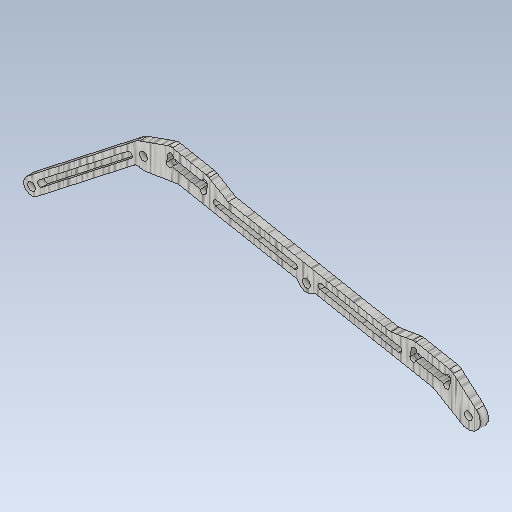
# Autodesk Inventor part: 台形サスバー２
Saved by Autodesk Inventor 2020 (Build 240168000, 168)
## iProperties
Created: 2019-11-14
Part Number: 台形サスバー２
Material: アルミニウム 7075
Document SubType Name: Modeling
Designer: tanjihayato
Density: 2.81 g/cm^3
Appearance: サテン - ブラシ仕上げ 重厚
Mass: 9.37217 g
Surface Area: 46.6831 cm^2
Volume: 3.33529 cm^3
Author: tanjihayato
Autodesk Inventor part; units mm, degrees
note: some values were not read from the file. Chosen so that the rebuilt part matches the saved one: sketch regions of "押し出し1".
ref_plane "YZ Plane" through (0, 0, 0) normal (1, 0, 0) x (0, 1, 0)
ref_plane "XZ Plane" through (0, 0, 0) normal (0, 1, 0) x (-1, 0, 0)
ref_plane "XY Plane" through (0, 0, 0) normal (0, 0, 1) x (1, 0, 0)
sketch "スケッチ1" plane through (0, 0, 0) normal (0, 0, 1) x (1, 0, 0)
  circle A0 centre (127.64315, 30.26217) radius 1.5
  circle A1 centre (5.936242, 53.5882) radius 1.5
  line L0 (5.936242, 53.5882) -> (127.64315, 30.26217) construction
  circle A2 centre (5.936242, 53.5882) radius 4.025
  circle A3 centre (127.64315, 30.26217) radius 4.025
  arc A4 (127.25169, 23.248085) -> (128.965476, 37.161596) centre (127.64315, 30.26217) ccw
  line L1 (12.835668, 52.265874) -> (13.400362, 55.212248)
  line L2 (15.462824, 54.816962) -> (26.069771, 52.784062)
  line L3 (28.132233, 52.388776) -> (27.567538, 49.442402)
  line L4 (14.89813, 51.870588) -> (25.505076, 49.837688)
  line L5 (120.743724, 31.584496) -> (121.308418, 34.53087)
  line L6 (119.245956, 34.926156) -> (108.63901, 36.959056)
  line L7 (106.576548, 37.354342) -> (106.011853, 34.407968)
  line L8 (108.074315, 34.012682) -> (118.681262, 31.979782)
  circle A5 centre (19.354562, 46.434577) radius 3
  circle A6 centre (112.530747, 28.576671) radius 3
  line L9 (7.258568, 60.487626) -> (128.965476, 37.161596)
  arc A7 (17.926333, 42.16724) -> (21.546529, 42.504529) centre (19.354562, 46.434577) ccw
  arc A8 (109.041036, 25.735559) -> (112.27999, 24.083663) centre (112.530747, 28.576671) ccw
  line L10 (3.706619, 46.926413) -> (17.926333, 42.16724)
  line L11 (112.27999, 24.083663) -> (127.25169, 23.248085)
  circle A9 centre (19.354562, 46.434577) radius 1.5
  circle A10 centre (112.530747, 28.576671) radius 1.5
  line L12 (32.344248, 48.52691) -> (21.546529, 42.504529)
  line L13 (109.041036, 25.735559) -> (101.235144, 35.32346)
  line L14 (32.344248, 48.52691) -> (101.235144, 35.32346)
  arc A11 (108.63901, 36.959056) -> (106.576548, 37.354342) centre (107.607779, 37.156699) ccw
  arc A12 (106.011853, 34.407968) -> (108.074315, 34.012682) centre (107.043084, 34.210325) ccw
  arc A13 (121.308418, 34.53087) -> (119.245956, 34.926156) centre (120.277187, 34.728513) ccw
  arc A14 (118.681262, 31.979782) -> (120.743724, 31.584496) centre (119.712493, 31.782139) ccw
  arc A15 (28.132233, 52.388776) -> (26.069771, 52.784062) centre (27.101002, 52.586419) ccw
  arc A16 (25.505076, 49.837688) -> (27.567538, 49.442402) centre (26.536307, 49.640045) ccw
  arc A17 (15.462824, 54.816962) -> (13.400362, 55.212248) centre (14.431593, 55.014605) ccw
  arc A18 (12.835668, 52.265874) -> (14.89813, 51.870588) centre (13.866899, 52.068231) ccw
  line L15 (5.936242, 53.5882) -> (-35.940425, 22.842004) construction
  circle A19 centre (-35.940425, 22.842004) radius 1.5
  arc A20 (-37.715892, 25.26021) -> (-34.164958, 20.423799) centre (-35.940425, 22.842004) ccw
  line L16 (-37.715892, 25.26021) -> (-0.959545, 52.247024)
  line L17 (-34.164958, 20.423799) -> (2.591389, 47.410613)
  arc A21 (7.258568, 60.487626) -> (-0.959545, 52.247024) centre (5.936242, 53.5882) ccw
  arc A22 (2.591389, 47.410613) -> (3.706619, 46.926413) centre (5.936242, 53.5882) ccw
  point P0 (0, 0)
  point P1 (0, 0)
  dimension "d0" = 8.05
  dimension "d1" = 8.05
  dimension "d2" = 3
  dimension "d3" = 3
  dimension "d4" = 15
  dimension "d5" = 3
  dimension "d6" = 15
  dimension "d7" = 6
  dimension "d8" = 6
  dimension "d9" = 9
  dimension "d10" = 9
  dimension "d11" = 3
  dimension "d12" = 3
  dimension "d13" = 7.5
  dimension "d14" = 7.5
  dimension "d15" = 40
  dimension "d16" = 40
  dimension "d17" = 2.1
  dimension "d18" = 2.1
  dimension "d19" = 2.1
  dimension "d20" = 2.1
  dimension "d21" = 2.1
  dimension "d22" = 2.1
  dimension "d23" = 2.1
  dimension "d24" = 2.1
  dimension "d25" = 3
  dimension "d26" = 6
  dimension "d27" = 3
  dimension "d28" = 3
  constraints: 36 end point, 28 point on circle, 23 centre point, 22 tangent, 14 point on line, 8 coincident, 4 parallel, 4 perpendicular, 1 collinear
  measures "d0" diameter of A2
  measures "d1" diameter of A3
  measures "d2" radial gap between concentric circles of A3 A4
  measures "d3" distance of L1.start L1.end
  measures "d4" distance of L1.end L3.start
  measures "d5" distance of L5.start L5.end
  measures "d6" distance of L5.end L7.start
  measures "d7" diameter of A5
  measures "d8" diameter of A6
  measures "d9" diameter of A7
  measures "d10" diameter of A8
  measures "d11" diameter of A9
  measures "d12" diameter of A10
  measures "d13" distance from line of A5.centre L3
  measures "d14" distance from line of A10.centre L7
  measures "d15" angle of L13 L0
  measures "d16" angle of L0 L12
  measures "d17" diameter of A11
  measures "d18" diameter of A12
  measures "d19" diameter of A13
  measures "d20" diameter of A14
  measures "d21" diameter of A15
  measures "d22" diameter of A16
  measures "d23" diameter of A17
  measures "d24" diameter of A18
  measures "d25" diameter of A19
  measures "d26" diameter of A20
  measures "d27" radial gap between concentric circles of A21 A2
  measures "d28" radial gap between concentric circles of A22 A2
sketch "スケッチ3" plane through (0, 0, 0) normal (0, 0, 1) x (1, 0, 0)
  circle A0 centre (0, 0) radius 10.1 construction
  circle A1 centre (25.320198, -9.936175) radius 17.1 construction
  circle A2 centre (110.474331, -16.4118) radius 28.1 construction
  circle A3 centre (62.413099, -12.756939) radius 20.1 construction
  circle A4 centre (-21.690847, -16.4118) radius 17.1 construction
  circle A5 centre (-105.525669, -16.4118) radius 28.1 construction
  line L0 (-170.91498, -81.4118) -> (490.004419, -81.4118)
  line L1 (-105.525669, -16.4118) -> (-21.690847, -16.4118) construction
  line L2 (110.474331, -16.4118) -> (25.320198, -9.936175) construction
  line L3 (110.474331, -16.4118) -> (104.150058, -0.631953)
  line L4 (104.150058, -0.631953) -> (95.593688, 20.717252) construction
  line L5 (95.593688, 20.717252) -> (70.474331, -10.4118) construction
  line L6 (70.474331, -10.4118) -> (110.474331, -16.4118) construction
  line L7 (-137.681852, 53.5882) -> (165.818568, 53.5882)
  line L8 (25.320198, -9.936175) -> (108.686903, 8.5882) construction
  line L9 (25.320198, -9.936175) -> (102.538646, -46.4118) construction
  line L10 (25.320198, -9.936175) -> (5.936242, 53.5882) construction
  line L11 (5.936242, 53.5882) -> (127.64315, 30.26217)
  line L12 (127.64315, 30.26217) -> (110.474331, -16.4118) construction
  line L13 (102.538646, -46.4118) -> (118.068109, 0.832921) construction
  line L14 (118.068109, 0.832921) -> (5.936242, 53.5882) construction
  line L15 (108.686903, 8.5882) -> (129.858294, 53.5882) construction
  line L16 (129.858294, 53.5882) -> (5.936242, 53.5882) construction
  line L17 (119.272599, 31.0882) -> (366.444098, 68.5882) construction
  line L18 (119.05874, 6.925185) -> (362.021337, 65.824902) construction
  line L19 (110.303378, -22.78944) -> (351.062397, 44.553669) construction
  line L20 (127.64315, 30.26217) -> (4.192658, 19.461651) construction
  circle A6 centre (80.474331, 23.123973) radius 3 construction
  circle A7 centre (80.474331, 23.123973) radius 1.5
  arc A8 (79.800999, 27.573313) -> (76.161969, 24.409872) centre (80.474331, 23.123973) ccw
  circle A9 centre (70.474331, -10.4118) radius 1.5
  arc A10 (66.161969, -9.125901) -> (69.424217, -14.787558) centre (70.474331, -10.4118) ccw
  circle A11 centre (150.474331, 0.5882) radius 1.5
  arc A12 (152.562257, -3.398097) -> (154.040845, 3.33228) centre (150.474331, 0.5882) ccw
  circle A13 centre (127.64315, 30.26217) radius 1.5
  arc A14 (131.281576, 32.91016) -> (126.969818, 34.71151) centre (127.64315, 30.26217) ccw
  circle A15 centre (110.474331, -16.4118) radius 5
  arc A16 (108.607462, -24.190926) -> (114.186199, -23.49855) centre (110.474331, -16.4118) ccw
  line L21 (76.161969, 24.409872) -> (66.161969, -9.125901)
  line L22 (69.424217, -14.787558) -> (108.607462, -24.190926)
  line L23 (114.186199, -23.49855) -> (152.562257, -3.398097)
  line L24 (154.040845, 3.33228) -> (131.209664, 33.00625)
  line L25 (126.969818, 34.71151) -> (79.800999, 27.573313)
  circle A17 centre (-145.525669, 0.5882) radius 1.5
  arc A18 (-149.092184, 3.33228) -> (-147.613596, -3.398097) centre (-145.525669, 0.5882) ccw
  circle A19 centre (-105.525669, -16.4118) radius 5
  arc A20 (-109.237538, -23.49855) -> (-103.6588, -24.190926) centre (-105.525669, -16.4118) ccw
  circle A21 centre (-65.525669, -10.4118) radius 1.5
  arc A22 (-64.475556, -14.787558) -> (-61.213308, -9.125901) centre (-65.525669, -10.4118) ccw
  circle A23 centre (0, 0) radius 20.05 construction
  circle A24 centre (110.474331, -16.4118) radius 30.1 construction
  circle A25 centre (62.413099, -12.756939) radius 22.1 construction
  circle A26 centre (25.320198, -9.936175) radius 19.1 construction
  circle A27 centre (0, 0) radius 12.1 construction
  circle A28 centre (-21.690847, -16.4118) radius 19.1 construction
  circle A29 centre (-105.525669, -16.4118) radius 30.1 construction
  circle A30 centre (0, 0) radius 20.55 construction
  circle A31 centre (95.593688, 20.717252) radius 4.025 construction
  circle A32 centre (95.593688, 20.717252) radius 6.025 construction
  circle A33 centre (-75.525669, 23.123973) radius 1.5
  arc A34 (-71.213308, 24.409872) -> (-74.852338, 27.573313) centre (-75.525669, 23.123973) ccw
  circle A35 centre (-122.694488, 30.26217) radius 1.5
  arc A36 (-122.021157, 34.71151) -> (-126.261003, 33.00625) centre (-122.694488, 30.26217) ccw
  line L26 (-126.261003, 33.00625) -> (-149.092184, 3.33228)
  line L27 (-147.613596, -3.398097) -> (-109.237538, -23.49855)
  line L28 (-103.6588, -24.190926) -> (-64.475556, -14.787558)
  line L29 (-61.213308, -9.125901) -> (-71.213308, 24.409872)
  line L30 (-74.852338, 27.573313) -> (-122.021157, 34.71151)
  circle A37 centre (14, -17.4118) radius 2.29213 construction
  circle A38 centre (-14, -17.4118) radius 2.29213 construction
  circle A39 centre (-14, -17.4118) radius 14 construction
  circle A40 centre (14, -17.4118) radius 14 construction
  line L31 (-170.651239, -31.4118) -> (202.86558, -31.4118)
  line L32 (5.936242, 53.5882) -> (-42.252867, 34.177029) construction
  line L33 (5.936242, 53.5882) -> (-29.404465, 15.509095) construction
  circle A41 centre (5.936242, 53.5882) radius 1.5
  arc A42 (9.961109, 55.600773) -> (4.254869, 57.762285) centre (5.936242, 53.5882) ccw
  line L34 (-21.690847, -16.4118) -> (-99.974162, 13.5882) construction
  line L35 (-21.690847, -16.4118) -> (-101.711328, -41.4118) construction
  line L36 (9.961109, 55.600773) -> (31.415648, 12.694659)
  circle A43 centre (-50.601037, 30.814282) radius 1.5
  arc A44 (-52.28241, 34.988367) -> (-54.424801, 28.441767) centre (-50.601037, 30.814282) ccw
  line L37 (4.254869, 57.762285) -> (-52.28241, 34.988367)
  line L38 (-54.424801, 28.441767) -> (-46.715132, 16.016156)
  circle A45 centre (27.390781, 10.682087) radius 3 construction
  circle A46 centre (-84.86606, 5.271327) radius 4.5 construction
  circle A47 centre (-132.017427, -1.981251) radius 4.5 construction
  line L39 (-132.701548, 2.466443) -> (-85.550181, 9.71902) construction
  arc A48 (26.900287, 6.208898) -> (31.415648, 12.694659) centre (27.390781, 10.682087) ccw
  arc A49 (-46.715132, 16.016156) -> (-43.381863, 13.915483) centre (-42.891368, 18.388671) ccw
  line L40 (-43.381863, 13.915483) -> (26.900287, 6.208898)
  circle A50 centre (-42.252867, 34.177029) radius 3 construction
  circle A51 centre (25.320198, -9.936175) radius 4.025 construction
  circle A52 centre (-21.690847, -16.4118) radius 4.025 construction
  circle A53 centre (-42.891368, 18.388671) radius 1.5
  circle A54 centre (27.390781, 10.682087) radius 1.5
  circle A55 centre (-57.813011, 39.770535) radius 4.5 construction
  circle A56 centre (-99.303951, 63.315241) radius 4.5 construction
  line L41 (5.936242, 53.5882) -> (-35.940425, 22.842004) construction
  circle A57 centre (-58.005574, -24.479052) radius 20.1 construction
  circle A58 centre (-58.005574, -24.479052) radius 22.1 construction
  line L42 (-53.326057, 39.428119) -> (-56.279689, 0.724331) construction
  circle A59 centre (-42.252867, 34.177029) radius 4.5
  dimension "d14" = 7.5
  dimension "d125" = 9
  dimension "d126" = 9
  dimension "d141" = 9
  dimension "d37" = 20.2
  dimension "d38" = 34.2
  dimension "d39" = 56.2
  dimension "d40" = 40.2
  dimension "d41" = 216
  dimension "d42" = 65
  dimension "d43" = 65
  dimension "d44" = 34.2
  dimension "d45" = 56.2
  dimension "d46" = 17
  dimension "d47" = 23
  dimension "d48" = 40
  dimension "d49" = 40
  dimension "d50" = 6
  dimension "d51" = 135
  dimension "d52" = 25
  dimension "d53" = 30
  dimension "d54" = 5
  dimension "d55" = 2
  dimension "d56" = 250
  dimension "d57" = 150
  dimension "d58" = 250
  dimension "d59" = 250
  dimension "d60" = 123.823
  dimension "d61" = 123.823
  dimension "d62" = 123.823
  dimension "d63" = 6
  dimension "d64" = 3
  dimension "d65" = 9
  dimension "d66" = 3
  dimension "d67" = 9
  dimension "d68" = 3
  dimension "d69" = 9
  dimension "d70" = 40
  dimension "d71" = 17
  dimension "d72" = 3
  dimension "d73" = 9
  dimension "d74" = 10
  dimension "d75" = 3
  dimension "d76" = 3
  dimension "d77" = 9
  dimension "d78" = 40
  dimension "d79" = 17
  dimension "d80" = 10
  dimension "d81" = 3
  dimension "d82" = 3
  dimension "d83" = 9
  dimension "d84" = 40
  dimension "d85" = 6
  dimension "d86" = 40.1
  dimension "d87" = 2
  dimension "d88" = 2
  dimension "d89" = 2
  dimension "d90" = 2
  dimension "d91" = 2
  dimension "d92" = 2
  dimension "d93" = 0.5
  dimension "d94" = 8.05
  dimension "d95" = 2
  dimension "d96" = 3
  dimension "d97" = 9
  dimension "d98" = 3
  dimension "d99" = 9
  dimension "d100" = 46.67397
  constraints: 86 end point, 57 centre point, 39 tangent, 29 coincident, 29 point on circle, 11 equal length, 5 horizontal, 3 midpoint, 3 point on line, 2 equal radius, 1 collinear, 1 parallel, 1 perpendicular, 13 other
  measures "d37" diameter of A0
  measures "d38" diameter of A1
  measures "d39" diameter of A2
  measures "d40" diameter of A3
  measures "d41" distance of L1.start L2.start
  measures "d42" distance from line of L0 L2.start
  measures "d43" distance from line of L0 L1.start
  measures "d44" diameter of A4
  measures "d45" diameter of A5
  measures "d46" distance of L2.start L3.end
  measures "d47" distance of L3.end L4.end
  measures "d48" distance of L4.end L5.end
  measures "d49" horizontal distance of L5.end L2.start
  measures "d50" vertical distance of L5.end L2.start
  measures "d51" distance between parallel lines of L0 L7
  measures "d52" vertical distance of L2.start L8.end
  measures "d53" vertical distance of L9.end L2.start
  measures "d54" angle of L12 L15
  measures "d55" angle of L12 L13
  measures "d56" distance of L17.start L17.end
  measures "d57" distance from line of L0 L17.end
  measures "d58" distance of L18.start L18.end
  measures "d59" distance of L19.start L19.end
  measures "d60" angle of L15 L17
  measures "d61" angle of L12 L18
  measures "d62" angle of L13 L19
  measures "d63" diameter of A6
  measures "d64" diameter of A7
  measures "d65" diameter of A8
  measures "d66" diameter of A9
  measures "d67" diameter of A10
  measures "d68" diameter of A11
  measures "d69" diameter of A12
  measures "d70" horizontal distance of L2.start A11.centre
  measures "d71" vertical distance of L2.start A11.centre
  measures "d72" diameter of A13
  measures "d73" diameter of A14
  measures "d74" diameter of A15
  measures "d75" radial gap between concentric circles of A15 A16
  measures "d76" diameter of A17
  measures "d77" diameter of A18
  measures "d78" horizontal distance of L1.start A17.centre
  measures "d79" vertical distance of L1.start A18.centre
  measures "d80" diameter of A19
  measures "d81" radial gap between concentric circles of A19 A20
  measures "d82" diameter of A21
  measures "d83" diameter of A22
  measures "d84" horizontal distance of L1.start A21.centre
  measures "d85" vertical distance of L1.start A21.centre
  measures "d86" diameter of A23
  measures "d87" radial gap between concentric circles of A2 A24
  measures "d88" radial gap between concentric circles of A3 A25
  measures "d89" radial gap between concentric circles of A1 A26
  measures "d90" radial gap between concentric circles of A0 A27
  measures "d91" radial gap between concentric circles of A4 A28
  measures "d92" radial gap between concentric circles of A5 A29
  measures "d93" radial gap between concentric circles of A23 A30
  measures "d94" diameter of A31
  measures "d95" radial gap between concentric circles of A31 A32
  measures "d96" diameter of A33
  measures "d97" diameter of A34
  measures "d98" diameter of A35
  measures "d99" diameter of A36
  measures "d100" vertical distance of L2.start L11.end
sketch "スケッチ2" plane through (0, 0, 0) normal (0, 0, 1) x (1, 0, 0)
  circle A0 centre (-35.940425, 22.842004) radius 1.5
  circle A1 centre (5.936242, 53.5882) radius 1.5
  circle A2 centre (127.64315, 30.26217) radius 1.5
  line L0 (19.061011, 51.072741) -> (114.518381, 32.777629)
  circle A3 centre (5.936242, 53.5882) radius 4.5
  circle A4 centre (127.64315, 30.26217) radius 4.5
  circle A5 centre (-35.940425, 22.842004) radius 3
  line L1 (5.0892, 49.168639) -> (6.071325, 48.980408)
  line L2 (6.071325, 48.980408) -> (19.061011, 51.072741)
  line L3 (114.518381, 32.777629) -> (125.813983, 26.03084)
  line L4 (125.813983, 26.03084) -> (126.796108, 25.842609)
  line L5 (4.441871, 57.832827) -> (15.204741, 61.622021)
  line L6 (-37.784972, 25.207939) -> (3.169421, 57.137102)
  line L7 (3.512579, 49.796649) -> (-34.095878, 20.47607)
  line L8 (122.00181, 41.153572) -> (130.601007, 33.653494)
  circle A6 centre (80.318062, 36.277771) radius 3
  circle A7 centre (80.318062, 36.277771) radius 4.5
  line L9 (128.210589, 34.72625) -> (80.885502, 40.741852)
  circle A8 centre (80.474331, 23.123973) radius 1.5
  line L10 (120.463576, 35.710991) -> (121.028271, 38.657365)
  line L11 (15.186361, 58.942751) -> (14.621667, 55.996377)
  circle A9 centre (66.977927, 42.90731) radius 1.5
  circle A10 centre (66.977927, 42.90731) radius 3
  line L12 (29.918232, 56.119279) -> (29.353537, 53.172905)
  arc A11 (17.248823, 58.547465) -> (15.186361, 58.942751) centre (16.217592, 58.745108) ccw
  arc A12 (29.918232, 56.119279) -> (27.85577, 56.514565) centre (28.887001, 56.316922) ccw
  arc A13 (27.291076, 53.568191) -> (29.353537, 53.172905) centre (28.322307, 53.370548) ccw
  arc A14 (14.621667, 55.996377) -> (16.684129, 55.601091) centre (15.652898, 55.798734) ccw
  line L13 (17.248823, 58.547465) -> (27.85577, 56.514565)
  line L14 (16.684129, 55.601091) -> (27.291076, 53.568191)
  arc A15 (31.882481, 55.742816) -> (27.00191, 58.714615) centre (28.887001, 56.316922) ccw
  line L15 (27.00191, 58.714615) -> (18.855609, 60.275914)
  arc A16 (18.855609, 60.275914) -> (15.204741, 61.622021) centre (16.217592, 58.745108) ccw
  line L16 (106.2964, 41.480837) -> (105.731706, 38.534463)
  arc A17 (108.358862, 41.085551) -> (106.2964, 41.480837) centre (107.327631, 41.283194) ccw
  arc A18 (121.028271, 38.657365) -> (118.965809, 39.052651) centre (119.99704, 38.855008) ccw
  arc A19 (118.401114, 36.106277) -> (120.463576, 35.710991) centre (119.432345, 35.908634) ccw
  arc A20 (105.731706, 38.534463) -> (107.794168, 38.139177) centre (106.762937, 38.33682) ccw
  line L17 (31.882481, 55.742816) -> (104.332151, 41.8573)
  line L18 (108.358862, 41.085551) -> (118.965809, 39.052651)
  line L19 (107.794168, 38.139177) -> (118.401114, 36.106277)
  arc A21 (122.00181, 41.153572) -> (118.111949, 41.252701) centre (119.99704, 38.855008) ccw
  line L20 (118.111949, 41.252701) -> (109.965648, 42.814)
  arc A22 (109.965648, 42.814) -> (104.332151, 41.8573) centre (107.327631, 41.283194) ccw
  line L21 (30.450999, 58.935397) -> (37.645199, 54.638348)
  line L22 (16.791698, 61.740588) -> (29.461109, 59.312402)
  line L23 (120.571146, 41.850488) -> (107.901737, 44.278674)
  line L24 (106.8426, 44.294381) -> (98.569433, 42.961768)
  point P0 (0, 0)
  dimension "d36" = 9
  dimension "d29" = 9
  dimension "d30" = 9
  dimension "d31" = 6
  dimension "d35" = 6
  dimension "d155" = 47.70588
  dimension "d156" = 47.70588
  dimension "d163" = 3
  dimension "d164" = 3
  dimension "d166" = 8.07688
  dimension "d167" = 8.07688
  dimension "d168" = 3
  dimension "d169" = 6
  dimension "d170" = 61.9691
  dimension "d171" = 61.9691
  dimension "d174" = 15
  dimension "d175" = 2.1
  dimension "d176" = 2
  dimension "d178" = 2
  dimension "d179" = 2
  dimension "d180" = 15
  dimension "d181" = 2.1
  dimension "d182" = 7
  dimension "d183" = 2
  dimension "d184" = 2
  dimension "d187" = 160
  dimension "d188" = 160
  dimension "d189" = 160
  dimension "d190" = 160
  dimension "d191" = 1
  dimension "d192" = 1
  constraints: 50 end point, 39 point on circle, 26 tangent, 18 centre point, 13 point on line, 9 perpendicular, 7 parallel, 6 equal radius, 5 coincident, 2 collinear, 5 other
  measures "d29" diameter of A3
  measures "d30" diameter of A4
  measures "d31" diameter of A5
  measures "d35" diameter of A6
  measures "d155" distance of A8.centre A2.centre
  measures "d156" distance of A2.centre A6.centre
  measures "d163" distance of L10.start L10.end
  measures "d164" distance of L11.start L11.end
  measures "d166" distance from line of A2.centre L10
  measures "d167" distance from line of A1.centre L11
  measures "d168" diameter of A9
  measures "d169" diameter of A10
  measures "d170" distance of A2.centre A9.centre
  measures "d171" distance of A1.centre A9.centre
  measures "d174" distance of L12.start L11.start
  measures "d175" diameter of A11
  measures "d176" distance between parallel lines of L13 L15
  measures "d178" radial gap between concentric circles of A11 A16
  measures "d179" radial gap between concentric circles of A12 A15
  measures "d180" distance of L10.end L16.start
  measures "d181" diameter of A17
  measures "d182" distance between parallel lines of L0 L17
  measures "d183" distance between parallel lines of L18 L20
  measures "d184" radial gap between concentric circles of A21 A18
  measures "d187" angle of L4 L3
  measures "d188" angle of L1 L2
  measures "d189" angle of L21 L17
  measures "d190" angle of L17 L24
  measures "d191" distance of L1.start L1.end
  measures "d192" distance of L3.end L4.end
extrude "押し出し1" add sketch "スケッチ2" along normal blind 3 contours L2 L1 A3 L5 A16 L15 A15 L17 A22 L20 A21 L8 A4 L9 L10 A18 L18 A17 L16 A20 A7 L0 A10 | A10 L0 A9 | L0 A9 A10 | A9 L0 | A3 | A7 L0 | L7 A5 L6 A3 | L9 A20 A19 A4 L4 L3 L0 A7 | A5 | A20 L19 A19 L9 | L22 A15 L15 A16 | A4 | L21 L17 A15 | L24 A22 L17 | A21 L20 A22 L23 picked at (66.846156, 43.480469) picked at (82.873228, 39.071854)
extrude "押し出し2" cut sketch "スケッチ2" along normal blind 3 contours A9 L0 | L0 A9
fillet "フィレット1" radius 2 1 edges at (3.5126, 49.7966, 1.5)
fillet "フィレット2" radius 2 2 edges at (64.0118, 42.4576, 1.5) (69.5676, 41.3928, 1.5)
sketch "スケッチ4" plane through (0, 0, 3) normal (0, 0, 1) x (1, 0, 0)
  circle A0 centre (66.977927, 42.90731) radius 1.5
  arc A1 (118.401114, 36.106277) -> (120.463576, 35.710991) centre (119.432345, 35.908634) ccw
  line L0 (118.401114, 36.106277) -> (107.794168, 38.139177)
  arc A2 (105.731706, 38.534463) -> (107.794168, 38.139177) centre (106.762937, 38.33682) ccw
  line L1 (105.731706, 38.534463) -> (106.2964, 41.480837)
  arc A3 (108.358862, 41.085551) -> (106.2964, 41.480837) centre (107.327631, 41.283194) ccw
  line L2 (108.358862, 41.085551) -> (118.965809, 39.052651)
  arc A4 (121.028271, 38.657365) -> (118.965809, 39.052651) centre (119.99704, 38.855008) ccw
  line L3 (121.028271, 38.657365) -> (120.463576, 35.710991)
  arc A5 (17.248823, 58.547465) -> (15.186361, 58.942751) centre (16.217592, 58.745108) ccw
  line L4 (17.248823, 58.547465) -> (27.85577, 56.514565)
  arc A6 (29.918232, 56.119279) -> (27.85577, 56.514565) centre (28.887001, 56.316922) ccw
  line L5 (29.918232, 56.119279) -> (29.353537, 53.172905)
  arc A7 (27.291076, 53.568191) -> (29.353537, 53.172905) centre (28.322307, 53.370548) ccw
  line L6 (27.291076, 53.568191) -> (16.684129, 55.601091)
  arc A8 (14.621667, 55.996377) -> (16.684129, 55.601091) centre (15.652898, 55.798734) ccw
  line L7 (14.621667, 55.996377) -> (15.186361, 58.942751)
  circle A9 centre (127.64315, 30.26217) radius 1.5
  circle A10 centre (5.936242, 53.5882) radius 1.5
  circle A11 centre (-35.940425, 22.842004) radius 1.5
  line L8 (-34.095878, 20.47607) -> (2.53893, 49.037566)
  arc A12 (4.435586, 49.345791) -> (2.53893, 49.037566) centre (3.768628, 47.460276) ccw
  arc A13 (4.435586, 49.345791) -> (5.0892, 49.168639) centre (5.936242, 53.5882) ccw
  line L9 (5.0892, 49.168639) -> (6.071325, 48.980408)
  line L10 (6.071325, 48.980408) -> (19.061011, 51.072741)
  line L11 (19.061011, 51.072741) -> (62.861197, 42.678111)
  arc A14 (64.282011, 41.591241) -> (62.861197, 42.678111) centre (62.484734, 40.713862) ccw
  arc A15 (64.282011, 41.591241) -> (68.99621, 40.68773) centre (66.977927, 42.90731) ccw
  arc A16 (70.718195, 41.172259) -> (68.99621, 40.68773) centre (70.341732, 39.20801) ccw
  line L12 (70.718195, 41.172259) -> (114.518381, 32.777629)
  line L13 (114.518381, 32.777629) -> (125.813983, 26.03084)
  line L14 (125.813983, 26.03084) -> (126.796108, 25.842609)
  arc A17 (126.796108, 25.842609) -> (130.601007, 33.653494) centre (127.64315, 30.26217) ccw
  line L15 (130.601007, 33.653494) -> (122.00181, 41.153572)
  arc A18 (122.00181, 41.153572) -> (120.571146, 41.850488) centre (119.99704, 38.855008) ccw
  line L16 (120.571146, 41.850488) -> (107.901737, 44.278674)
  arc A19 (107.901737, 44.278674) -> (106.8426, 44.294381) centre (107.327631, 41.283194) ccw
  line L17 (106.8426, 44.294381) -> (98.569433, 42.961768)
  line L18 (98.569433, 42.961768) -> (37.645199, 54.638348)
  line L19 (37.645199, 54.638348) -> (30.450999, 58.935397)
  arc A20 (30.450999, 58.935397) -> (29.461109, 59.312402) centre (28.887001, 56.316922) ccw
  line L20 (29.461109, 59.312402) -> (16.791698, 61.740588)
  arc A21 (16.791698, 61.740588) -> (15.204741, 61.622021) centre (16.217592, 58.745108) ccw
  line L21 (15.204741, 61.622021) -> (4.441871, 57.832827)
  arc A22 (4.441871, 57.832827) -> (3.169421, 57.137102) centre (5.936242, 53.5882) ccw
  line L22 (3.169421, 57.137102) -> (-37.784972, 25.207939)
  arc A23 (-37.784972, 25.207939) -> (-34.095878, 20.47607) centre (-35.940425, 22.842004) ccw
  line L23 (-35.940425, 22.842004) -> (21.626177, 67.722498) construction
  line L24 (3.169421, 57.137102) -> (-37.784972, 25.207939)
  line L25 (-32.746413, 25.332143) -> (0.799881, 51.48575) construction
  line L26 (-32.100822, 24.504066) -> (1.445473, 50.657673)
  line L27 (0.15429, 52.313827) -> (-33.392005, 26.16022)
  arc A24 (-33.392005, 26.16022) -> (-32.100822, 24.504066) centre (-32.746413, 25.332143) ccw
  arc A25 (1.445473, 50.657673) -> (0.15429, 52.313827) centre (0.799881, 51.48575) ccw
  line L28 (-3.227881, 58.908275) -> (147.857843, 29.951576) construction
  line L29 (98.569433, 42.961768) -> (37.645199, 54.638348)
  line L30 (62.582031, 46.295317) -> (33.18792, 51.928916) construction
  line L31 (62.779674, 47.326548) -> (33.385564, 52.960147)
  line L32 (32.990277, 50.897685) -> (62.384388, 45.264087)
  arc A26 (62.384388, 45.264087) -> (62.779674, 47.326548) centre (62.582031, 46.295317) ccw
  arc A27 (33.385564, 52.960147) -> (32.990277, 50.897685) centre (33.18792, 51.928916) ccw
  line L33 (72.314981, 44.429926) -> (101.709091, 38.796327) construction
  line L34 (72.117338, 43.398695) -> (101.511448, 37.765096)
  line L35 (101.906734, 39.827557) -> (72.512624, 45.461156)
  arc A28 (72.512624, 45.461156) -> (72.117338, 43.398695) centre (72.314981, 44.429926) ccw
  arc A29 (101.511448, 37.765096) -> (101.906734, 39.827557) centre (101.709091, 38.796327) ccw
  circle A30 centre (66.977927, 42.90731) radius 4.5 construction
  point P0 (0, 0)
  point P1 (-15.973266, 38.408946)
  point P2 (47.884976, 49.112117)
  point P3 (87.012036, 41.613126)
  dimension "d195" = 2.1
  dimension "d196" = 3.5
  dimension "d197" = 3.5
  dimension "d198" = 2.1
  dimension "d199" = 2.1
  dimension "d200" = 4
  dimension "d201" = 4
  dimension "d204" = 9
  constraints: 28 end point, 16 tangent, 12 point on circle, 7 centre point, 5 midpoint, 5 parallel, 5 point on line, 1 coincident
  measures "d195" diameter of A25
  measures "d196" distance between parallel lines of L28 L18
  measures "d197" distance between parallel lines of L12 L28
  measures "d198" diameter of A27
  measures "d199" diameter of A29
  measures "d200" distance from line of L30.end L5
  measures "d201" distance from line of L33.end L1
  measures "d204" diameter of A30
extrude "押し出し3" cut sketch "スケッチ4" against normal blind 2.5 contours A24 L27 A25 L26 | A26 L32 A27 L31 | A28 L35 A29 L34
equation "\"d16\" = d15"
equation "\"d44\" = d38"
equation "\"d45\" = d39"
equation "\"d61\" = d60"
equation "\"d62\" = d60"
equation "\"d156\" = d155"
equation "\"d167\" = d166"
equation "\"d171\" = d170"
